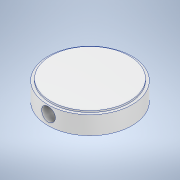
# Autodesk Inventor part: Platogrueso
Saved by Autodesk Inventor 2020.3 (Build 243373000, 373)
## iProperties
Created: 2020-06-17
Part Number: Platogrueso
Material: Aluminum 6061
Document SubType Name: Modeling
Designer: Juan
Density: 2.7 g/cm^3
Appearance: Aluminum - Flat
Author: Juan
Autodesk Inventor part; units mm, degrees
note: some values were not read from the file. Chosen so that the rebuilt part matches the saved one: direction of "Hole2".
ref_plane "YZ Plane" through (0, 0, 0) normal (1, 0, 0) x (0, 1, 0)
ref_plane "XZ Plane" through (0, 0, 0) normal (0, 1, 0) x (-1, 0, 0)
sketch "Sketch1" plane through (0, 0, 0) normal (0, 1, 0) x (-1, 0, 0)
  circle A0 centre (0, 0) radius 50.8
  dimension "d0" = 101.6
  constraints: 1 centre point, 1 coincident
  measures "d0" diameter of A0
extrude "Extrusion1" add sketch "Sketch1" along normal blind 24
ref_plane "Work Plane1" through (0, 0, 50.8) normal (0, 0, 1) x (1, 0, 0)
sketch "Sketch3" plane through (0, 0, 50.8) normal (0, 0, 1) x (1, 0, 0)
  line L0 (50.8, 24) -> (-50.8, 24) projected
  line L1 (0, 24) -> (0, 12) construction
  point P0 (0, 0)
  dimension "d7" = 12
  constraints: 2 end point, 1 midpoint, 1 vertical
  measures "d7" distance of L1.start L1.end
hole "Hole1" at (0, 12, 50.8) direction (0, 0, -1) diameter 16.5 depth 88.9 tip angle 118
sketch "Sketch4" plane through (0, 0, 0) normal (0, -1, 0) x (1, 0, 0)
  line L0 (0, 0) -> (0, -25) construction
  line L1 (0, 0) -> (0, 25) construction
  dimension "d15" = 25
  dimension "d16" = 25
  constraints: 4 end point, 2 vertical
  measures "d15" distance of L0.start L0.end
  measures "d16" distance of L0.start L1.end
hole "Hole2" at (0, 0, 25) at (0, 0, -25) direction (0, 1, 0) diameter 4.134 end up to surface thread size "M5x0.8" class "6H" standard "ANSI Metric M Profile"
sketch "Sketch5" plane through (0, 0, 0) normal (0, -1, 0) x (1, 0, 0)
  point P0 (0, 0)
  point P1 (-19.6272, 0)
hole "Hole3" at (-19.6272, 0, 0) direction (0, 1, 0) diameter 4.917 depth 12 tip angle 118 thread size "M6x1" class "6H" standard "ANSI Metric M Profile"
ref_plane "Work Plane2" through (0, 0, -38.1) normal (0, 0, 1) x (1, 0, 0)
sketch "Sketch7" plane through (0, 24, 0) normal (0, 1, 0) x (1, 0, 0)
  circle A0 centre (0, 0) radius 50.8
  circle A1 centre (0, 0) radius 47.5
  dimension "d35" = 101.6
  dimension "d36" = 95
  constraints: 2 centre point, 2 coincident
  measures "d35" diameter of A0
  measures "d36" diameter of A1
extrude "Extrusion4" cut sketch "Sketch7" against normal blind 2
body "Solid1"
